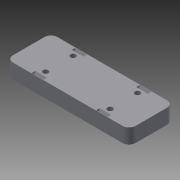
# Autodesk Inventor part: singleBaccable-ucan_fysect_CAP
Saved by Autodesk Inventor 2014 SP2 (Build 180246200, 246)
## iProperties
Created: 2025-01-14
Part Number: singleBaccable-ucan_fysect_CAP
Material: Generic
Document SubType Name: Sheet Metal
Designer: GauchoHP
Density: 1 g/cm^3
Sheet Metal Rule: Default_mm
Appearance: Default
Author: GauchoHP
Autodesk Inventor part; units mm, degrees
ref_plane "YZ Plane" through (0, 0, 0) normal (1, 0, 0) x (0, 1, 0)
ref_plane "XZ Plane" through (0, 0, 0) normal (0, 1, 0) x (-1, 0, 0)
ref_plane "XY Plane" through (0, 0, 0) normal (0, 0, 1) x (1, 0, 0)
sketch "Sketch1" plane through (0, 0, 0) normal (0, 0, 1) x (1, 0, 0)
  line L0 (-8.8921, 9.8249) -> (43.1079, 9.8249)
  line L1 (46.1079, 6.8249) -> (46.1079, -8.1751)
  line L2 (43.1079, -11.1751) -> (-8.8921, -11.1751)
  line L3 (-11.8921, -8.1751) -> (-11.8921, 6.8249)
  arc A0 (-8.8921, 9.8249) -> (-11.8921, 6.8249) centre (-8.8921, 6.8249) ccw
  arc A1 (46.1079, 6.8249) -> (43.1079, 9.8249) centre (43.1079, 6.8249) ccw
  arc A2 (43.1079, -11.1751) -> (46.1079, -8.1751) centre (43.1079, -8.1751) ccw
  arc A3 (-11.8921, -8.1751) -> (-8.8921, -11.1751) centre (-8.8921, -8.1751) ccw
  line L4 (43.1079, 7.8249) -> (-8.8921, 7.8249)
  arc A4 (-8.8921, 7.8249) -> (-9.8921, 6.8249) centre (-8.8921, 6.8249) ccw
  line L5 (-9.8921, 6.8249) -> (-9.8921, -8.1751)
  arc A5 (-9.8921, -8.1751) -> (-8.8921, -9.1751) centre (-8.8921, -8.1751) ccw
  line L6 (-8.8921, -9.1751) -> (43.1079, -9.1751)
  arc A6 (43.1079, -9.1751) -> (44.1079, -8.1751) centre (43.1079, -8.1751) ccw
  line L7 (44.1079, -8.1751) -> (44.1079, 6.8249)
  arc A7 (44.1079, 6.8249) -> (43.1079, 7.8249) centre (43.1079, 6.8249) ccw
  circle A8 centre (2.6079, -7.1751) radius 2.5
  circle A9 centre (2.6079, -7.1751) radius 1.25
  circle A10 centre (2.6079, 5.8249) radius 2.5
  circle A11 centre (2.6079, 5.8249) radius 1.25
  circle A12 centre (33.1079, 5.8249) radius 2.5
  circle A13 centre (33.1079, 5.8249) radius 1.25
  circle A14 centre (33.1079, -7.1751) radius 2.5
  circle A15 centre (33.1079, -7.1751) radius 1.25
  point P0 (0, 0)
  point P1 (-11.8921, 9.8249)
  point P2 (46.1079, 9.8249)
  point P3 (-11.8921, -11.1751)
  dimension "d0" = 58
  dimension "d1" = 21
  dimension "d2" = 3
  dimension "d5" = 2
  dimension "d6" = 5
  dimension "d7" = 2.5
  dimension "d8" = 5
  dimension "d9" = 2.5
  dimension "d10" = 5
  dimension "d11" = 2.5
  dimension "d12" = 5
  dimension "d13" = 2.5
  dimension "d14" = 30.5
  dimension "d15" = 30.5
  dimension "d16" = 13
  dimension "d17" = 2
  dimension "d18" = 11
  dimension "d19" = 11
  constraints: 16 centre point, 16 end point, 16 point on circle, 8 tangent, 6 point on line, 4 coincident, 4 parallel, 3 equal radius, 2 perpendicular, 1 horizontal, 7 other
  measures "d0" distance of point (-11.892, 9.825) point (46.108, 9.825)
  measures "d1" distance of point (-11.892, -11.175) point (-11.892, 9.825)
  measures "d2" radius of A0
  measures "d5" distance between parallel lines of L4 L0
  measures "d6" diameter of A8
  measures "d7" diameter of A9
  measures "d8" diameter of A10
  measures "d9" diameter of A11
  measures "d10" diameter of A12
  measures "d11" diameter of A13
  measures "d12" diameter of A14
  measures "d13" diameter of A15
  measures "d14" distance of A12.centre A10.centre
  measures "d15" distance of A14.centre A8.centre
  measures "d16" distance of A8.centre A10.centre
  measures "d17" distance from line of L6 A8.centre
  measures "d18" distance from line of L7 A12.centre
  measures "d19" distance from line of L7 A14.centre
extrude "Extrusion1" add sketch "Sketch1" along normal blind 7 contours L0 A1 L1 A2 L2 A3 L3 A0 | A12 L4 | L4 A12 | A10 L4 | L4 A10 | A14 L6 | L6 A14 | A8 L6 | L6 A8
sketch "Sketch2" plane through (0, 0, 7) normal (0, 0, 1) x (1, 0, 0)
  circle A0 centre (2.6079, 5.8249) radius 1.25 projected
  line L0 (43.1079, 9.8249) -> (-8.8921, 9.8249) projected
  line L1 (-8.8921, -11.1751) -> (43.1079, -11.1751) projected
  circle A1 centre (33.1079, -7.1751) radius 1.25 projected
  circle A2 centre (33.1079, 5.8249) radius 1.25 projected
  circle A3 centre (2.6079, -7.1751) radius 1.25 projected
  line L2 (-0.1421, 9.1749) -> (5.3579, 9.1749)
  line L3 (5.3579, 9.1749) -> (5.3579, 8.4749)
  line L4 (5.3579, 8.4749) -> (-0.1421, 8.4749)
  line L5 (-0.1421, 8.4749) -> (-0.1421, 9.1749)
  line L6 (35.8579, 9.1749) -> (30.3579, 9.1749)
  line L7 (30.3579, 9.1749) -> (30.3579, 8.4749)
  line L8 (30.3579, 8.4749) -> (35.8579, 8.4749)
  line L9 (35.8579, 8.4749) -> (35.8579, 9.1749)
  line L10 (30.3579, -9.8251) -> (35.8579, -9.8251)
  line L11 (35.8579, -9.8251) -> (35.8579, -10.5251)
  line L12 (35.8579, -10.5251) -> (30.3579, -10.5251)
  line L13 (30.3579, -10.5251) -> (30.3579, -9.8251)
  line L14 (-0.1421, -9.8251) -> (5.3579, -9.8251)
  line L15 (5.3579, -9.8251) -> (5.3579, -10.5251)
  line L16 (5.3579, -10.5251) -> (-0.1421, -10.5251)
  line L17 (-0.1421, -10.5251) -> (-0.1421, -9.8251)
  point P0 (0, 0)
  dimension "d20" = 5.5
  dimension "d21" = 0.7
  dimension "d22" = 0.65
  dimension "d23" = 2.75
  dimension "d24" = 0.7
  dimension "d25" = 0.65
  dimension "d27" = 5.5
  dimension "d29" = 2.75
  dimension "d30" = 5.5
  dimension "d31" = 0.7
  dimension "d32" = 0.65
  dimension "d33" = 2.75
  dimension "d34" = 0.7
  dimension "d35" = 5.5
  dimension "d36" = 2.75
  dimension "d37" = 0.65
  constraints: 32 end point, 8 parallel, 4 horizontal, 4 perpendicular
  measures "d20" distance of L2.start L2.end
  measures "d21" distance of L2.end L3.end
  measures "d22" distance between parallel lines of L0 L2
  measures "d23" distance from line of L3 A0.centre
  measures "d24" distance of L6.end L7.end
  measures "d25" distance between parallel lines of L0 L6
  measures "d27" distance of L6.start L6.end
  measures "d29" distance from line of L7 A2.centre
  measures "d30" distance of L10.start L10.end
  measures "d31" distance of L10.end L11.end
  measures "d32" distance between parallel lines of L1 L12
  measures "d33" distance from line of L13 A1.centre
  measures "d34" distance of L14.end L15.end
  measures "d35" distance of L14.start L14.end
  measures "d36" distance from line of L17 A3.centre
  measures "d37" distance between parallel lines of L1 L16
extrude "Extrusion2" cut sketch "Sketch2" against normal blind 1.2 contours L2 L3 L4 L5 | L9 L8 L7 L6 | L10 L11 L12 L13 | L14 L15 L16 L17
chamfer "Chamfer1" distance 0.5 distance2 1.2 1 edges at (2.6079, -9.8251, 7) measured on face at (2.6079, -9.3251, 7)
chamfer "Chamfer2" distance 0.5 distance2 1.2 1 edges at (2.6079, -10.5251, 7) measured on face at (2.6079, -10.6251, 7)
chamfer "Chamfer3" distance 0.5 distance2 1.2 1 edges at (33.1079, -9.8251, 7) measured on face at (33.1079, -9.3251, 7)
chamfer "Chamfer4" distance 0.5 distance2 1.2 1 edges at (33.1079, -10.5251, 7) measured on face at (33.1079, -10.6251, 7)
chamfer "Chamfer5" distance 0.5 distance2 1.2 1 edges at (33.1079, 8.4749, 7) measured on face at (33.1079, 7.9749, 7)
chamfer "Chamfer6" distance 0.5 distance2 1.2 1 edges at (33.1079, 9.1749, 7) measured on face at (33.1079, 9.6749, 7)
chamfer "Chamfer7" distance 0.5 distance2 1.2 1 edges at (2.6079, 8.4749, 7) measured on face at (2.6079, 7.9749, 7)
chamfer "Chamfer8" distance 0.5 distance2 1.2 1 edges at (2.6079, 9.1749, 7) measured on face at (2.6079, 9.6749, 7)
sketch "Sketch3" plane through (0, 0, 0) normal (0, 0, -1) x (-1, 0, 0)
  circle A0 centre (-2.6079, -7.1751) radius 1.25
  line L0 (-43.1079, -11.1751) -> (8.8921, -11.1751)
  line L1 (8.8921, 9.8249) -> (-43.1079, 9.8249)
  circle A1 centre (-33.1079, 5.8249) radius 1.25
  circle A2 centre (-33.1079, -7.1751) radius 1.25
  circle A3 centre (-2.6079, 5.8249) radius 1.25
  line L2 (0.1421, -10.5251) -> (-5.3579, -10.5251)
  line L3 (-5.3579, -10.5251) -> (-5.3579, -9.8251)
  line L4 (-5.3579, -9.8251) -> (0.1421, -9.8251)
  line L5 (0.1421, -9.8251) -> (0.1421, -10.5251)
  line L6 (-35.8579, -10.5251) -> (-30.3579, -10.5251)
  line L7 (-30.3579, -10.5251) -> (-30.3579, -9.8251)
  line L8 (-30.3579, -9.8251) -> (-35.8579, -9.8251)
  line L9 (-35.8579, -9.8251) -> (-35.8579, -10.5251)
  line L10 (-30.3579, 8.4749) -> (-35.8579, 8.4749)
  line L11 (-35.8579, 8.4749) -> (-35.8579, 9.1749)
  line L12 (-35.8579, 9.1749) -> (-30.3579, 9.1749)
  line L13 (-30.3579, 9.1749) -> (-30.3579, 8.4749)
  line L14 (0.1421, 8.4749) -> (-5.3579, 8.4749)
  line L15 (-5.3579, 8.4749) -> (-5.3579, 9.1749)
  line L16 (-5.3579, 9.1749) -> (0.1421, 9.1749)
  line L17 (0.1421, 9.1749) -> (0.1421, 8.4749)
  point P0 (0, 0)
  point P1 (0, -1.3503)
  dimension "d64" = 5.5
  dimension "d65" = 0.7
  dimension "d66" = 0.65
  dimension "d67" = 2.75
  dimension "d68" = 0.7
  dimension "d69" = 0.65
  dimension "d70" = 5.5
  dimension "d71" = 2.75
  dimension "d72" = 5.5
  dimension "d73" = 0.7
  dimension "d74" = 0.65
  dimension "d75" = 2.75
  dimension "d76" = 0.7
  dimension "d77" = 5.5
  dimension "d78" = 2.75
  dimension "d79" = 0.65
  constraints: 36 end point, 8 parallel, 4 centre point, 4 perpendicular
  measures "d64" distance of L2.start L2.end
  measures "d65" distance of L2.end L3.end
  measures "d66" distance between parallel lines of L0 L2
  measures "d67" distance from line of L3 A0.centre
  measures "d68" distance of L6.end L7.end
  measures "d69" distance between parallel lines of L0 L6
  measures "d70" distance of L6.start L6.end
  measures "d71" distance from line of L7 A2.centre
  measures "d72" distance of L10.start L10.end
  measures "d73" distance of L10.end L11.end
  measures "d74" distance between parallel lines of L1 L12
  measures "d75" distance from line of L13 A1.centre
  measures "d76" distance of L14.end L15.end
  measures "d77" distance of L14.start L14.end
  measures "d78" distance from line of L17 A3.centre
  measures "d79" distance between parallel lines of L1 L16
extrude "Extrusion3" cut sketch "Sketch3" against normal blind 1.2 contours L2 L3 L4 L5 | L9 L8 L7 L6 | L10 L11 L12 L13 | L14 L15 L16 L17
chamfer "Chamfer9" distance 0.5 distance2 1.2 1 edges at (33.1079, 8.4749, 0) measured on face at (33.1079, 7.9749, 0)
chamfer "Chamfer10" distance 0.5 distance2 1.2 1 edges at (33.1079, 9.1749, 0) measured on face at (33.1079, 9.6749, 0)
chamfer "Chamfer11" distance 0.5 distance2 1.2 1 edges at (33.1079, -10.5251, 0) measured on face at (33.1079, -11.0251, 0)
chamfer "Chamfer12" distance 0.5 distance2 1.2 1 edges at (33.1079, -9.8251, 0) measured on face at (33.1079, -9.3251, 0)
chamfer "Chamfer13" distance 0.5 distance2 1.2 1 edges at (2.6079, 9.1749, 0) measured on face at (2.6079, 9.2749, 0)
chamfer "Chamfer14" distance 0.5 distance2 1.2 1 edges at (2.6079, 8.4749, 0) measured on face at (2.6079, 7.9749, 0)
chamfer "Chamfer15" distance 0.5 distance2 1.2 1 edges at (2.6079, -9.8251, 0) measured on face at (2.6079, -9.3251, 0)
chamfer "Chamfer16" distance 0.5 distance2 1.2 1 edges at (2.6079, -10.5251, 0) measured on face at (2.6079, -10.6251, 0)
sketch "Sketch5" plane through (0, 0, 7) normal (0, 0, 1) x (1, 0, 0)
  arc A0 (4.1079, -9.1751) -> (1.1079, -9.1751) centre (2.6079, -7.1751) ccw projected
  line L0 (1.1079, -9.1751) -> (-8.8921, -9.1751) projected
  arc A1 (-9.8921, -8.1751) -> (-8.8921, -9.1751) centre (-8.8921, -8.1751) ccw projected
  line L1 (-9.8921, -8.1751) -> (-9.8921, 6.8249) projected
  arc A2 (-8.8921, 7.8249) -> (-9.8921, 6.8249) centre (-8.8921, 6.8249) ccw projected
  line L2 (-8.8921, 7.8249) -> (1.1079, 7.8249) projected
  arc A3 (1.1079, 7.8249) -> (4.1079, 7.8249) centre (2.6079, 5.8249) ccw projected
  line L3 (4.1079, 7.8249) -> (31.6079, 7.8249) projected
  arc A4 (31.6079, 7.8249) -> (34.6079, 7.8249) centre (33.1079, 5.8249) ccw projected
  line L4 (34.6079, 7.8249) -> (43.1079, 7.8249) projected
  arc A5 (44.1079, 6.8249) -> (43.1079, 7.8249) centre (43.1079, 6.8249) ccw projected
  line L5 (44.1079, 6.8249) -> (44.1079, -8.1751) projected
  arc A6 (43.1079, -9.1751) -> (44.1079, -8.1751) centre (43.1079, -8.1751) ccw projected
  line L6 (43.1079, -9.1751) -> (34.6079, -9.1751) projected
  arc A7 (34.6079, -9.1751) -> (31.6079, -9.1751) centre (33.1079, -7.1751) ccw projected
  line L7 (31.6079, -9.1751) -> (4.1079, -9.1751) projected
  point P0 (0, 0)
extrude "Extrusion5" add sketch "Sketch5" against normal blind 2
equation "\"BendRadius\" = Thickness"
equation "\"BendReliefWidth\" = Thickness"
equation "\"BendReliefDepth\" = 0.5 * Thickness"
equation "\"CornerReliefSize\" = 4 * Thickness"
equation "\"MinimumRemnant\" = 2 * Thickness"
equation "\"TransitionRadius\" = BendRadius"
equation "\"JacobiRadiusSize\" = BendRadius"
equation "\"GapSize\" = Thickness"
equation "\"Thickness\" = 0.5"
body "Solid1"
